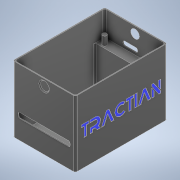
# Autodesk Inventor part: Case - Base
Saved by Autodesk Inventor 2021 (Build 250183000, 183)
## iProperties
Created: 2023-01-24
Part Number: Case - Base
Material: Plástico PC/ABS
Document SubType Name: Modeling
Designer: nicho
Density: 0.357273 g/cm^3
Appearance: Liso - Preto
Author: nicho
Autodesk Inventor part; units mm, degrees
ref_plane "YZ Plane" through (0, 0, 0) normal (1, 0, 0) x (0, 1, 0)
ref_plane "XZ Plane" through (0, 0, 0) normal (0, 1, 0) x (-1, 0, 0)
ref_plane "XY Plane" through (0, 0, 0) normal (0, 0, 1) x (1, 0, 0)
sketch "Esboço1" plane through (0, 0, 0) normal (0, 1, 0) x (-1, 0, 0)
  line L0 (-50, -26.5) -> (50, -26.5)
  line L1 (50, -26.5) -> (50, 26.5)
  line L2 (50, 26.5) -> (-50, 26.5)
  line L3 (-50, 26.5) -> (-50, -26.5)
  line L4 (-50, -26.5) -> (50, 26.5) construction
  line L5 (50, -26.5) -> (-50, 26.5) construction
  point P0 (0, 0)
  dimension "d0" = 100
  dimension "d1" = 53
  constraints: 12 end point, 2 midpoint, 2 parallel, 1 horizontal, 1 perpendicular
  measures "d0" distance of L2.end L1.end
  measures "d1" distance of L1.end L0.end
extrude "Extrusão1" add sketch "Esboço1" along normal blind 30
sketch "Esboço2" plane through (0, 30, 0) normal (0, 1, 0) x (1, 0, 0)
  line L0 (-50, 26.5) -> (-50, -26.5) projected
  line L1 (-50, -26.5) -> (50, -26.5) projected
  line L2 (50, -26.5) -> (50, 26.5) projected
  line L3 (50, 26.5) -> (-50, 26.5) projected
  line L4 (-49.5, -26) -> (-49.5, 26)
  line L5 (-49.5, 26) -> (49.5, 26)
  line L6 (49.5, 26) -> (49.5, -26)
  line L7 (49.5, -26) -> (-49.5, -26)
  point P0 (0, 0)
  dimension "d4" = 0.5
  constraints: 8 end point, 3 other
  measures "d4" distance between parallel lines of L0 L4
extrude "Extrusão2" cut sketch "Esboço2" against normal blind 29.5 contours L4 L5 L6 L7
sketch "Esboço3" plane through (50, 0, -26.5) normal (0, 0, -1) x (-1, 0, 0)
  line L0 (89, 27.5) -> (80.5, 27.5)
  line L1 (80.5, 27.5) -> (80.5, 25)
  line L2 (80.5, 25) -> (89, 25)
  line L3 (89, 25) -> (89, 27.5)
  line L4 (100, 0) -> (100, 30) projected
  line L5 (0, 30) -> (100, 30) projected
  point P0 (50, 0)
  dimension "d7" = 11
  dimension "d8" = 19.5
  dimension "d9" = 2.5
  dimension "d10" = 2.5
  constraints: 8 end point, 2 parallel, 1 horizontal, 1 perpendicular
  measures "d7" distance between parallel lines of L4 L3
  measures "d8" distance between parallel lines of L4 L1
  measures "d9" distance between parallel lines of L0 L2
  measures "d10" distance between parallel lines of L5 L0
extrude "Extrusão3" cut sketch "Esboço3" against normal up to surface (52.5 mm away)
fillet "Arredondamento1" radius 1 4 edges at (-39, 25, -26.25) (-39, 27.5, -26.25) (-30.5, 27.5, -26.25) (-30.5, 25, -26.25)
sketch "Esboço4" plane through (0, 0.5, 0) normal (0, 1, 0) x (1, 0, 0)
  line L0 (-49.5, 26) -> (49.5, 26) projected
  line L1 (-49.5, 26) -> (-18, 26)
  line L2 (-18, 26) -> (-18, 20.5)
  line L3 (-18, 20.5) -> (-49.5, 20.5)
  line L4 (-49.5, 20.5) -> (-49.5, 26)
  point P0 (0, 0)
  dimension "d15" = 5.5
  dimension "d16" = 31.5
  constraints: 8 end point, 2 parallel, 1 horizontal, 1 perpendicular
  measures "d15" distance of L1.end L2.end
  measures "d16" distance of L2.end L3.end
extrude "Extrusão4" add sketch "Esboço4" along normal blind 23
sketch "Esboço5" plane through (0, 23.5, 0) normal (0, 1, 0) x (1, 0, 0)
  circle A0 centre (-46.079, 22.5) radius 1.25
  line L0 (-49.5, -26) -> (-49.5, 26) projected
  line L1 (-49.5, 26) -> (49.5, 26) projected
  circle A1 centre (-21.579, 22.5) radius 1.25
  point P0 (0, 0)
  dimension "d19" = 3.421
  dimension "d20" = 3.5
  dimension "d21" = 2.5
  dimension "d22" = 2.5
  dimension "d23" = 24.5
  constraints: 2 centre point, 1 horizontal alignment
  measures "d19" distance from line of L0 A0.centre
  measures "d20" distance from line of L1 A0.centre
  measures "d21" diameter of A0
  measures "d22" diameter of A1
  measures "d23" distance of A1.centre A0.centre
extrude "Extrusão5" add sketch "Esboço5" along normal blind 5
sketch "Esboço6" plane through (-50, 0, 26.5) normal (0, 0, 1) x (1, 0, 0)
  line L0 (3, 11) -> (33, 11)
  line L1 (33, 11) -> (33, 14)
  line L2 (33, 14) -> (3, 14)
  line L3 (3, 14) -> (3, 11)
  line L4 (0, 0) -> (100, 0) projected
  line L5 (0, 0) -> (0, 30) projected
  point P0 (50, 0)
  dimension "d26" = 11
  dimension "d27" = 14
  dimension "d28" = 30
  dimension "d29" = 3
  constraints: 8 end point, 2 parallel, 1 horizontal, 1 perpendicular
  measures "d26" distance between parallel lines of L0 L4
  measures "d27" distance between parallel lines of L4 L2
  measures "d28" distance of L0.start L0.end
  measures "d29" distance between parallel lines of L5 L3
extrude "Extrusão6" cut sketch "Esboço6" against normal up to surface (47 mm away)
sketch "Esboço7" plane through (-50, 0, 26.5) normal (0, 0, 1) x (1, 0, 0)
  line L0 (0, 30) -> (100, 30) projected
  line L1 (100, 30) -> (36, 30)
  line L2 (36, 30) -> (36, 0)
  line L3 (36, 0) -> (100, 0)
  line L4 (100, 0) -> (100, 30)
  line L5 (33, 14) -> (33, 11) projected
  point P0 (50, 0)
  point P1 (36, 30)
  dimension "d32" = 3
  constraints: 8 end point, 2 parallel, 1 coincident, 1 horizontal, 1 perpendicular
  measures "d32" distance between parallel lines of L5 L2
extrude "Extrusão7" cut sketch "Esboço7" against normal up to surface (53 mm away)
sketch "Esboço8" plane through (0, 0.5, 0) normal (0, 1, 0) x (1, 0, 0)
  line L0 (-14.5, 26) -> (-14.5, -26)
  line L1 (-14, -26) -> (-14, 26) projected
  line L2 (-14, -26) -> (-49.5, -26) projected
  line L3 (-49.5, 26) -> (-14, 26) projected
  point P0 (0, 0)
  dimension "d35" = 0.5
  constraints: 2 end point, 2 point on line, 1 vertical alignment
  measures "d35" distance between parallel lines of L1 L0
extrude "Extrusão8" add sketch "Esboço8" along normal up to surface (29.5 mm away)
fillet "Arredondamento3" radius 1 11 edges at (-14, 15, 26.5) (-14, 15, -26.5) (-49.5, 12, -20.5) (-49.5, 26.75, -26) (-49.5, 15.25, 26) (-50, 15, -26.5) (-14.5, 15.25, 26) (-50, 15, 26.5) (-14.5, 15.25, -26) (-18, 12, -20.5) (-18, 12, -26)
fillet "Arredondamento4" radius 1 4 edges at (-47, 11, 26.25) (-47, 14, 26.25) (-17, 14, 26.25) (-17, 11, 26.25)
sketch "Esboço9" plane through (0, 30, 0) normal (0, 1, 0) x (1, 0, 0)
  arc A0 (-50, -25.5) -> (-49, -26.5) centre (-49, -25.5) ccw projected
  line L0 (-49, -26.5) -> (-15, -26.5) projected
  arc A1 (-15, -26.5) -> (-14, -25.5) centre (-15, -25.5) ccw projected
  line L1 (-14, 25.5) -> (-14, -25.5) projected
  arc A2 (-14, 25.5) -> (-15, 26.5) centre (-15, 25.5) ccw projected
  line L2 (-15, 26.5) -> (-49, 26.5) projected
  arc A3 (-49, 26.5) -> (-50, 25.5) centre (-49, 25.5) ccw projected
  line L3 (-50, 25.5) -> (-50, -25.5) projected
  arc A4 (-15.5, -26) -> (-14.5, -25) centre (-15.5, -25) ccw projected
  line L4 (-15.5, -26) -> (-48.5, -26) projected
  arc A5 (-49.5, -25) -> (-48.5, -26) centre (-48.5, -25) ccw projected
  line L5 (-49.5, -25) -> (-49.5, 25) projected
  arc A6 (-48.5, 26) -> (-49.5, 25) centre (-48.5, 25) ccw projected
  line L6 (-48.5, 26) -> (-15.5, 26) projected
  arc A7 (-14.5, 25) -> (-15.5, 26) centre (-15.5, 25) ccw projected
  line L7 (-14.5, -25) -> (-14.5, 25) projected
  point P0 (0, 0)
extrude "Extrusão9" add sketch "Esboço9" along normal blind 8
sketch "Esboço10" plane through (-49, 0, 26.5) normal (0, 0, 1) x (1, 0, 0)
  line L0 (0, 38) -> (34, 38) projected
  point P0 (49, 0)
  point P1 (17, 34)
  point P2 (17, 38)
  dimension "d42" = 4
  constraints: 1 midpoint, 1 vertical alignment
  measures "d42" distance from line of L0 point (17, 34)
hole "Furo1" at (-32, 34, 26.5) direction (0, 0, -1) diameter 3 depth 0.5 countersink diameter 6 countersink angle 90
sketch "Esboço11" plane through (-15, 0, -26.5) normal (0, 0, -1) x (-1, 0, 0)
  circle A0 centre (17, 34) radius 2.5 projected
  point P0 (-15, 0)
  dimension "d13" = 1
  constraints: 1 coincident
hole "Furo2" at (-32, 34, -26.5) direction (0, 0, 1) diameter 3 depth 0.5 countersink diameter 6 countersink angle 90
sketch "Esboço12" plane through (-14, 0, 25.5) normal (1, 0, 0) x (0, 0, -1)
  line L0 (4.064, 15) -> (4.064, 20.5)
  line L1 (4.064, 20.5) -> (2.564, 20.5)
  line L2 (2.564, 20.5) -> (2.564, 22)
  line L3 (2.564, 22) -> (7.064, 22)
  line L4 (7.064, 22) -> (7.064, 20.5)
  line L5 (7.064, 20.5) -> (5.564, 20.5)
  line L6 (5.564, 20.5) -> (5.564, 15)
  line L7 (5.564, 15) -> (4.064, 15)
  line L8 (51, 0) -> (0, 0) projected
  line L9 (0, 0) -> (0, 38) projected
  line L10 (7.564, 22) -> (10.564, 22)
  line L11 (7.564, 20.5) -> (10.564, 20.5)
  line L12 (7.564, 15) -> (7.564, 18)
  line L13 (7.564, 15) -> (9.064, 15)
  line L14 (9.064, 15) -> (9.064, 16.5)
  line L15 (9.064, 16.5) -> (10.564, 16.5)
  line L16 (10.564, 16.5) -> (11.7387, 15)
  line L17 (10.564, 16.5) -> (12.4693, 16.5) construction
  line L18 (11.7387, 15) -> (13.644, 15)
  line L19 (13.644, 15) -> (12.4693, 16.5)
  line L20 (7.564, 18) -> (10.564, 18)
  circle A0 centre (10.564, 18.92) radius 3.08
  circle A1 centre (10.564, 19.25) radius 1.25
  line L21 (7.564, 20.5) -> (7.564, 22)
  line L22 (14.144, 15) -> (17.0153, 22)
  line L23 (17.0153, 22) -> (18.5153, 22)
  line L24 (18.5153, 22) -> (21.3866, 15)
  line L25 (21.3866, 15) -> (19.7653, 15)
  line L26 (19.7653, 15) -> (17.7653, 19.8759)
  line L27 (17.7653, 19.8759) -> (15.7653, 15)
  line L28 (15.7653, 15) -> (14.144, 15)
  circle A2 centre (25.3866, 18.5) radius 3.5
  circle A3 centre (25.3866, 18.5) radius 2
  line L29 (25.3866, 18.5) -> (27.8614, 16.0251)
  line L30 (25.3866, 18.5) -> (27.8614, 20.9749)
  line L31 (25.3866, 18.5) -> (28.8866, 18.5)
  line L32 (29.8614, 15) -> (31.3614, 15)
  line L33 (31.3614, 15) -> (31.3614, 20.5)
  line L34 (31.3614, 20.5) -> (32.8614, 20.5)
  line L35 (32.8614, 20.5) -> (32.8614, 22)
  line L36 (32.8614, 22) -> (28.3614, 22)
  line L37 (28.3614, 22) -> (28.3614, 20.5)
  line L38 (28.3614, 20.5) -> (29.8614, 20.5)
  line L39 (29.8614, 20.5) -> (29.8614, 15)
  line L40 (33.3614, 22) -> (33.3614, 15)
  line L41 (33.3614, 15) -> (34.8614, 15)
  line L42 (34.8614, 15) -> (34.8614, 22)
  line L43 (34.8614, 22) -> (33.3614, 22)
  line L44 (35.3614, 15) -> (38.2327, 22)
  line L45 (38.2327, 22) -> (39.7327, 22)
  line L46 (47, 0.5) -> (47, 23.5) projected
  line L47 (39.7327, 22) -> (42.604, 15)
  line L48 (42.604, 15) -> (40.9827, 15)
  line L49 (40.9827, 15) -> (38.9827, 19.8759)
  line L50 (38.9827, 19.8759) -> (36.9827, 15)
  line L51 (36.9827, 15) -> (35.3614, 15)
  line L52 (46, 0.5) -> (46, 23.5) projected
  line L53 (43.104, 15) -> (44.604, 15)
  line L54 (43.104, 15) -> (43.104, 20.1283)
  line L55 (43.104, 20.1283) -> (44.604, 17.9861)
  line L56 (44.604, 17.9861) -> (44.604, 15)
  line L57 (43.104, 21) -> (43.104, 22)
  line L58 (43.104, 22) -> (44.235, 22)
  line L59 (44.235, 22) -> (48.4362, 16)
  line L60 (48.4362, 16) -> (48.4362, 15)
  line L61 (48.4362, 15) -> (47.3053, 15)
  line L62 (47.3053, 15) -> (43.104, 21)
  line L63 (48.4362, 16.8717) -> (48.4362, 22)
  line L64 (48.4362, 22) -> (46.9362, 22)
  line L65 (46.9362, 22) -> (46.9362, 19.0139)
  line L66 (46.9362, 19.0139) -> (48.4362, 16.8717)
  point P0 (25.5, 0)
  point P1 (13.644, 18.92)
  point P2 (25.3866, 15)
  point P3 (21.8866, 18.5)
  point P4 (26.8008, 19.9142)
  point P5 (26.8008, 17.0858)
  point P6 (12.4693, 16.5)
  dimension "d57" = 1.5
  dimension "d58" = 1.5
  dimension "d59" = 1.5
  dimension "d60" = 1.5
  dimension "d61" = 5.5
  dimension "d62" = 15
  dimension "d64" = 0.5
  dimension "d65" = 3
  dimension "d66" = 3
  dimension "d67" = 1.5
  dimension "d68" = 1.5
  dimension "d71" = 1.5
  dimension "d72" = 3
  dimension "d73" = 1.5
  dimension "d74" = 1.5
  dimension "d75" = 1.5
  dimension "d76" = 0.5
  dimension "d80" = 4
  dimension "d81" = 2
  dimension "d82" = 7
  dimension "d83" = 0.5
  dimension "d84" = 1.5
  dimension "d85" = 90
  dimension "d86" = 45
  dimension "d87" = 1.5
  dimension "d89" = 1.5
  dimension "d90" = 1.5
  dimension "d91" = 1.5
  dimension "d92" = 1.5
  dimension "d94" = 0.5
  dimension "d95" = 1.5
  dimension "d96" = 0.5
  dimension "d97" = 1.5
  dimension "d98" = 4
  dimension "d99" = 2
  dimension "d100" = 1.5
  dimension "d101" = 1.5
  dimension "d102" = 0.5
  dimension "d103" = 0.5
  dimension "d104" = 1.5
  dimension "d105" = 0.5
  dimension "d106" = 1.5
  dimension "d108" = 35
  dimension "d109" = 1.5
  dimension "d110" = 0.5
  dimension "d113" = 2.564
  dimension "d114" = 1
  dimension "d115" = 1
  constraints: 126 end point, 25 horizontal alignment, 20 perpendicular, 12 horizontal, 11 parallel, 8 point on circle, 8 vertical alignment, 7 vertical, 6 point on line, 3 centre point, 1 coincident, 1 collinear, 1 equal length, 1 tangent, 3 other
  measures "d57" distance of L6.end L0.start
  measures "d58" distance of L3.end L4.end
  measures "d59" distance of L0.end L1.end
  measures "d60" distance of L4.end L5.end
  measures "d61" distance between parallel lines of L7 L1
  measures "d62" distance between parallel lines of L8 L7
  measures "d64" distance of L3.end L10.start
  measures "d65" distance of L11.start L11.end
  measures "d66" distance of L12.start L12.end
  measures "d67" distance of L12.start L13.end
  measures "d68" distance of L13.end L14.end
  measures "d71" distance between parallel lines of L19 L16
  measures "d72" distance of L12.end L20.end
  measures "d73" distance between parallel lines of L22 L27
  measures "d74" distance between parallel lines of L24 L26
  measures "d75" distance of L22.end L23.end
  measures "d76" distance of L18.end L22.start
  measures "d80" distance of L27.end L25.end
  measures "d81" horizontal distance of L25.end L26.end
  measures "d82" diameter of A2
  measures "d83" horizontal distance of L24.end A2.end
  measures "d84" radial gap between concentric circles of A2 A3
  measures "d85" angle of L29 L30
  measures "d86" angle of L31 L30
  measures "d87" distance of L32.start L32.end
  measures "d89" distance of L33.end L34.end
  measures "d90" distance of L34.end L35.end
  measures "d91" distance of L36.end L37.end
  measures "d92" distance of L37.end L38.end
  measures "d94" distance from line of L37 L30.end
  measures "d95" distance of L42.end L40.start
  measures "d96" distance between parallel lines of L35 L40
  measures "d97" distance of L44.end L45.end
  measures "d98" distance of L48.end L50.end
  measures "d99" horizontal distance of L48.end L49.end
  measures "d100" distance between parallel lines of L44 L50
  measures "d101" distance between parallel lines of L47 L49
  measures "d102" distance of L41.end L44.start
  measures "d103" distance between parallel lines of L62 L55
  measures "d104" distance between parallel lines of L62 L59
  measures "d105" distance of L47.end L53.start
  measures "d106" distance of L53.start L53.end
  measures "d108" angle of L54 L55
  measures "d109" distance between parallel lines of L63 L65
  measures "d110" distance between parallel lines of L59 L66
  measures "d113" distance between parallel lines of L9 L2
  measures "d114" distance of L57.start L57.end
  measures "d115" distance of L59.end L60.end
extrude "Extrusão10" cut sketch "Esboço12" against normal blind 0.25 contours L0 L1 L2 L3 L4 L5 L6 L7 | L10 A0 L11 L21 | A0 L16 L15 L14 L20 A1 L11 | L19 L18 L16 A0 | A0 L14 L13 L12 L20 | L22 L23 L24 L25 L26 L27 L28 | L30 A3 L29 A2 | L39 L38 L37 L36 L35 L34 L33 L32 | L43 L42 L41 L40 | L44 L45 L47 L48 L49 L50 L51 | L62 L52 L59 L46 | L46 L59 L60 L61 L62 | L62 L57 L58 L59 L52 | L66 L65 L64 L46 | L46 L64 L63 L66 | L54 L55 L56 L53
